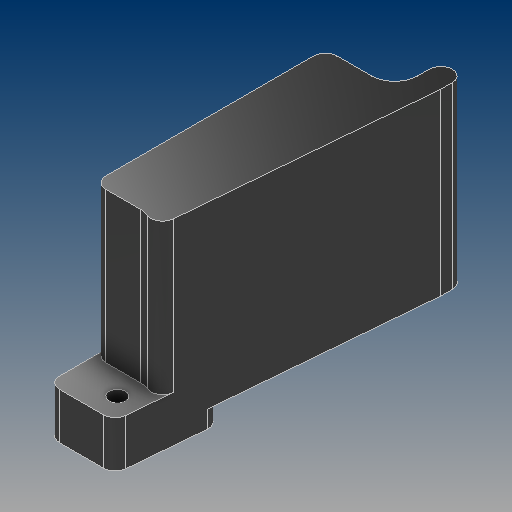
# Autodesk Inventor part: INtk_016_PelletDeflector1
Saved by Autodesk Inventor 2024.3 (Build 283343000, 343)
## iProperties
Created: 2024-08-07
Part Number: INtk_016_PelletDeflector1
Material: PC/ABS Plastic
Document SubType Name: Modeling
Designer: Kenji
Density: 1.1 g/cm^3
Appearance: Glossy - Black
Mass: 84.0825 g
Surface Area: 138.684 cm^2
Volume: 76.4386 cm^3
Author: Kenji
Autodesk Inventor part; units mm, degrees
ref_plane "YZ Plane" through (0, 0, 0) normal (1, 0, 0) x (0, 1, 0)
ref_plane "XZ Plane" through (0, 0, 0) normal (0, 1, 0) x (-1, 0, 0)
ref_plane "XY Plane" through (0, 0, 0) normal (0, 0, 1) x (1, 0, 0)
sketch "Sketch1" plane through (0, 0, 0) normal (0, 1, 0) x (-1, 0, 0)
  circle A0 centre (0, 0) radius 2.2479
  line L0 (0, 0) -> (0, 76.2) construction
  circle A1 centre (0, 76.2) radius 2.2479
  line L1 (9.525, 82.55) -> (-9.525, 82.55)
  line L2 (-12.7, 79.375) -> (-12.7, -3.175)
  line L3 (-9.525, -6.35) -> (9.525, -6.35)
  line L4 (12.7, -3.175) -> (12.7, 79.375)
  line L5 (0, 0) -> (0, 55.5752) construction
  line L6 (12.7, 55.5752) -> (-12.7, 55.5752) construction
  line L7 (12.7, 55.5752) -> (-12.7, 55.5752)
  arc A2 (12.7, 79.375) -> (9.525, 82.55) centre (9.525, 79.375) ccw
  arc A3 (-9.525, 82.55) -> (-12.7, 79.375) centre (-9.525, 79.375) ccw
  arc A4 (9.525, -6.35) -> (12.7, -3.175) centre (9.525, -3.175) ccw
  arc A5 (-12.7, -3.175) -> (-9.525, -6.35) centre (-9.525, -3.175) ccw
  point P0 (-12.7, -6.35)
  point P1 (12.7, -6.35)
  dimension "d0" = 4.4958
  dimension "d1" = 4.4958
  dimension "d2" = 76.2
  dimension "d3" = 25.4
  dimension "d4" = 12.7
  dimension "d5" = 6.35
  dimension "d6" = 6.35
  dimension "d7" = 55.5752
  dimension "d8" = 3.175
  constraints: 16 end point, 8 point on circle, 8 tangent, 7 point on line, 6 centre point, 3 equal radius, 3 parallel, 2 coincident, 2 perpendicular, 1 collinear, 1 horizontal, 1 midpoint, 1 vertical
  measures "d0" diameter of A0
  measures "d1" diameter of A1
  measures "d2" distance of L0.start L0.end
  measures "d3" distance of point (12.7, -6.35) point (-12.7, -6.35)
  measures "d4" distance between parallel lines of L0 L4
  measures "d5" distance from line of L1 A1.centre
  measures "d6" distance from line of L0.start L3
  measures "d7" distance of L0.start L5.end
  measures "d8" radius of A2
extrude "Extrusion1" add sketch "Sketch1" along normal blind 53.975
sketch "Sketch2" plane through (0, 53.975, 0) normal (0, 1, 0) x (1, 0, 0)
  line L0 (12.7, -79.375) -> (12.7, 3.175) projected
  arc A0 (12.7, 3.175) -> (9.525, 6.35) centre (9.525, 3.175) ccw projected
  line L1 (9.525, 6.35) -> (-9.525, 6.35) projected
  arc A1 (-9.525, 6.35) -> (-12.7, 3.175) centre (-9.525, 3.175) ccw projected
  line L2 (-12.7, 3.175) -> (-12.7, -79.375) projected
  arc A2 (-12.7, -79.375) -> (-9.525, -82.55) centre (-9.525, -79.375) ccw projected
  line L3 (-9.525, -82.55) -> (9.525, -82.55) projected
  arc A3 (9.525, -82.55) -> (12.7, -79.375) centre (9.525, -79.375) ccw projected
  circle A4 centre (0, 0) radius 2.2479 projected
  circle A5 centre (0, -76.2) radius 2.2479 projected
  line L4 (5.5044, -82.55) -> (12.7, 0)
  line L5 (12.7, -79.375) -> (12.7, 3.175) projected
  line L6 (-12.7, 0) -> (12.7, 0) construction
  line L7 (2.2479, -76.2) -> (6.0579, -76.2) construction
  line L8 (5.5044, -82.55) -> (12.7, -82.55)
  line L9 (12.7, -82.55) -> (12.7, 0)
  point P0 (12.7, 0)
  dimension "d14" = 3.81
  constraints: 10 end point, 7 point on line, 2 horizontal, 1 coincident, 1 horizontal alignment, 1 midpoint, 1 perpendicular, 1 vertical, 1 other
  measures "d14" distance of L7.start L7.end
extrude "Extrusion3" cut sketch "Sketch2" against normal through all contours A3 L3 L4 L0
fillet "Fillet2" radius 3.175 1 edges at (5.5044, 26.9875, 82.55)
sketch "Sketch3" plane through (0, 53.975, 0) normal (0, 1, 0) x (1, 0, 0)
  point P0 (0, 0)
extrude "Extrusion4" cut sketch "Sketch1" along normal blind 4.7752 contours L4 A4 L3 A5 L2 L7
fillet "Fillet3" radius 3.175 2 edges at (7.8557, 2.3876, 55.5752) (-12.7, 2.3876, 55.5752)
sketch "Sketch5" plane through (0, 53.975, 0) normal (0, 1, 0) x (1, 0, 0)
  circle A0 centre (0, -76.2) radius 2.2479 projected
  circle A1 centre (0, 0) radius 2.2479 projected
  arc A2 (2.5941, -82.55) -> (5.7571, -79.6507) centre (2.5941, -79.375) ccw projected
  line L0 (5.7571, -79.6507) -> (12.7, 0) projected
  line L1 (12.7, 0) -> (12.7, 3.175) projected
  arc A3 (12.7, 3.175) -> (9.525, 6.35) centre (9.525, 3.175) ccw projected
  line L2 (9.525, 6.35) -> (-9.525, 6.35) projected
  arc A4 (-9.525, 6.35) -> (-12.7, 3.175) centre (-9.525, 3.175) ccw projected
  line L3 (-12.7, 3.175) -> (-12.7, -79.375) projected
  arc A5 (-12.7, -79.375) -> (-9.525, -82.55) centre (-9.525, -79.375) ccw projected
  line L4 (-9.525, -82.55) -> (2.5941, -82.55) projected
  circle A6 centre (0, 0) radius 6.35 construction
  line L5 (6.35, 0) -> (6.35, 6.35)
  line L6 (0, -6.35) -> (-12.7, -6.35)
  arc A7 (0, -6.35) -> (6.35, 0) centre (0, 0) ccw
  line L7 (6.35, 6.35) -> (-12.7, 6.35)
  line L8 (-12.7, 6.35) -> (-12.7, -6.35)
  circle A8 centre (0, -76.2) radius 6.35 construction
  line L9 (0, -69.85) -> (-12.7, -69.85)
  line L10 (6.1837, -74.7564) -> (5.5044, -82.55)
  line L11 (5.5044, -82.55) -> (-12.7, -82.55)
  line L12 (-12.7, -82.55) -> (-12.7, -69.85)
  line L13 (-9.525, -82.55) -> (2.5941, -82.55) projected
  arc A9 (6.1837, -74.7564) -> (0, -69.85) centre (0, -76.2) ccw
  dimension "d21" = 12.7
  dimension "d22" = 12.7
  constraints: 16 end point, 8 point on circle, 6 point on line, 5 tangent, 4 centre point, 4 perpendicular, 2 coincident, 2 collinear, 1 concentric, 1 horizontal
  measures "d21" diameter of A6
  measures "d22" diameter of A8
extrude "Extrusion5" cut sketch "Sketch5" against normal blind 41.275 contours L4 A5 L3 L9 A9 L0 A2 | L3 A4 L2 L5 A7 L6
fillet "Fillet4" radius 3.175 1 edges at (6.1837, 33.3375, 74.7564)
fillet "Fillet5" radius 3.175 3 edges at (-12.7, 33.3375, 69.85) (-12.7, 33.3375, 6.35) (6.35, 33.3375, -6.35)
body "Solid1"
